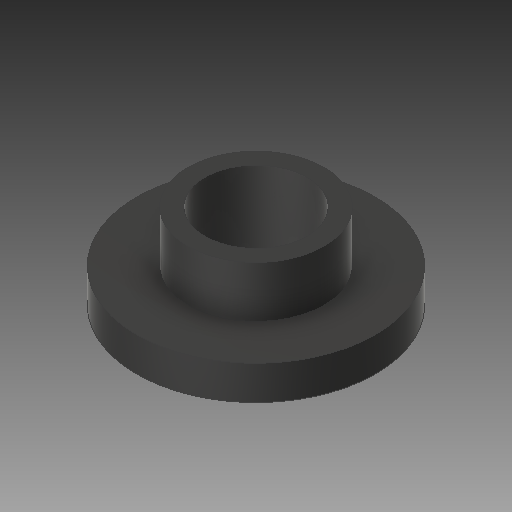
# Autodesk Inventor part: D3040-7815B
Saved by Autodesk Inventor 2018 (Build 220112000, 112)
## iProperties
Created: 2016-08-26
Part Number: D3040-7815B
Material: アセタール樹脂、黒
Document SubType Name: Modeling
Designer: hiro
Density: 1.425 g/cm^3
Appearance: 滑らか - 黒
Mass: 0.0565192 g
Surface Area: 1.27235 cm^2
Volume: 0.0396626 cm^3
Author: hiro
Autodesk Inventor part; units mm, degrees
ref_plane "YZ Plane" through (0, 0, 0) normal (1, 0, 0) x (0, 1, 0)
ref_plane "XZ Plane" through (0, 0, 0) normal (0, 1, 0) x (-1, 0, 0)
ref_plane "XY Plane" through (0, 0, 0) normal (0, 0, 1) x (1, 0, 0)
sketch "スケッチ1" plane through (0, 0, 0) normal (0, 0, 1) x (1, 0, 0)
  line L0 (1.5, 1.25) -> (1.5, -1.25)
  line L1 (1.5, -1.25) -> (3.5, -1.25)
  line L2 (3.5, -1.25) -> (3.5, -0.25)
  line L3 (3.5, -0.25) -> (2, -0.25)
  line L4 (2, -0.25) -> (2, 1.25)
  line L5 (2, 1.25) -> (1.5, 1.25)
  line L6 (0, 1.7364) -> (0, -1.7364) construction
  point P0 (0, 0)
  point P1 (0, 0)
  point P2 (1.5, 0)
  dimension "d0" = 3
  dimension "d1" = 4
  dimension "d2" = 1
  dimension "d3" = 1.5
  dimension "d4" = 7
  constraints: 14 end point, 4 perpendicular, 2 midpoint, 2 vertical, 1 coincident, 1 horizontal, 1 horizontal alignment
  measures "d0" diameter of L0 L6
  measures "d1" diameter of L4 L6
  measures "d2" distance of L1.end L2.end
  measures "d3" distance of L3.end L4.end
  measures "d4" diameter of L2 L6
revolve "回転1" add sketch "スケッチ1" angle 360 about axis through (0, 1.7364, 0) along (0, -1, 0)
